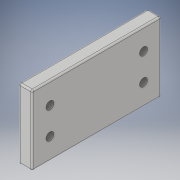
# Autodesk Inventor part: Clamp Plate V2
Saved by Autodesk Inventor 2019 (Build 230136000, 136)
## iProperties
Created: 2019-06-10
Part Number: Clamp Plate V2
Material: Generic
Document SubType Name: Modeling
Designer: Matthew XPS
Density: 1 g/cm^3
Appearance: Default
Author: Matthew XPS
Autodesk Inventor part; units mm, degrees
ref_plane "YZ Plane" through (0, 0, 0) normal (1, 0, 0) x (0, 1, 0)
ref_plane "XZ Plane" through (0, 0, 0) normal (0, 1, 0) x (-1, 0, 0)
ref_plane "XY Plane" through (0, 0, 0) normal (0, 0, 1) x (1, 0, 0)
sketch "Sketch1" plane through (0, 0, 0) normal (1, 0, 0) x (0, 1, 0)
  line L0 (-13, 24) -> (-13, -24)
  line L1 (-13, -24) -> (13, -24)
  line L2 (13, -24) -> (13, 24)
  line L3 (13, 24) -> (-13, 24)
  line L4 (-13, 24) -> (13, -24) construction
  line L5 (-13, -24) -> (13, 24) construction
  point P0 (0, 0)
  dimension "d0" = 48
  dimension "d1" = 26
  constraints: 12 end point, 2 midpoint, 2 parallel, 1 perpendicular, 1 vertical
  measures "d0" distance of L0.start L0.end
  measures "d1" distance of L1.end L0.end
extrude "Extrusion1" add sketch "Sketch1" along normal blind 5
sketch "Sketch2" plane through (5, 0, 0) normal (1, 0, 0) x (0, 0, -1)
  circle A0 centre (17.4055, -5) radius 1.5
  line L0 (3.065, 0) -> (34.1813, 0)
  circle A1 centre (17.4055, 5) radius 1.5
  point P0 (0, 0)
  dimension "d5" = 3
  dimension "d11" = 17.4055
  dimension "d12" = 5
  constraints: 2 centre point, 2 end point, 1 horizontal, 1 symmetric about line, 1 other
  measures "d5" diameter of A0
  measures "d11" horizontal distance of A0.centre point (0, 0)
  measures "d12" vertical distance of point (0, 0) A0.centre
extrude "Extrusion2" cut sketch "Sketch2" against normal blind 3 contours A0
thread "Thread1" size "M3x0.5" class "6H" standard "ANSI Metric M Profile" full length
mirror "Mirror1" about plane through (0, 0, 0) normal (0, 0, 1) of "Extrusion2"
fillet "Fillet1" radius 0.6 12 edges at (5, -13, 0) (0, -13, 0) (2.5, -13, -24) (5, 0, -24) (0, 0, -24) (2.5, 13, -24) (5, 13, 0) (0, 13, 0) (2.5, 13, 24) (5, 0, 24) (2.5, -13, 24) (0, 0, 24)
mirror "Mirror2" about plane through (0, 0, 0) normal (0, 1, 0) of "Extrusion2", "Mirror1"
body "Solid1"
